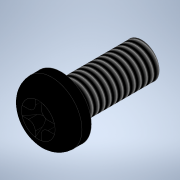
# Autodesk Inventor part: F-2606EB
Saved by Autodesk Inventor 2022.3 (Build 263350000, 350)
## iProperties
Part Number: F-2606EB
Material: チタン
Document SubType Name: Modeling
Designer: Masato Kubotera
Density: 6.22441 g/cm^3
Appearance: 陽極酸化 - 黒
Mass: 0.657 g
Surface Area: 1.94048 cm^2
Volume: 0.105552 cm^3
Description: ReadyMade
Catalog Web Link: https://wilco.jp/products/F/F-EB.html#page3
Author: Masato Kubotera
Autodesk Inventor part; units mm, degrees
ref_plane "YZ Plane" through (0, 0, 0) normal (1, 0, 0) x (0, 1, 0)
ref_plane "XZ Plane" through (0, 0, 0) normal (0, 1, 0) x (-1, 0, 0)
ref_plane "XY Plane" through (0, 0, 0) normal (0, 0, 1) x (1, 0, 0)
sketch "スケッチ1" plane through (0, 0, 0) normal (1, 0, 0) x (0, 1, 0)
  line L0 (0, 7.7) -> (0, 0)
  line L1 (0, 0) -> (1.25, 0)
  line L2 (2.25, 1) -> (2.25, 1.7)
  line L3 (2.25, 1.7) -> (1.3, 1.7)
  line L4 (1.3, 1.7) -> (1.3, 7.7)
  line L5 (1.3, 7.7) -> (0, 7.7)
  line L6 (1.25, 0) -> (0, 1.7)
  arc A0 (1.25, 0) -> (2.25, 1) centre (1.25, 1) ccw
  line L7 (1.25, 0) -> (2.25, 0)
  line L8 (2.25, 0) -> (2.25, 1)
  dimension "d2" = 1.7
  dimension "d10" = 6
  dimension "d11" = 2.6
  dimension "d12" = 4.5
  dimension "d14" = 1
  constraints: 18 end point, 6 perpendicular, 4 point on line, 2 point on circle, 2 tangent, 1 centre point, 1 horizontal, 1 vertical
  measures "d2" distance of L7.end L2.end
  measures "d10" distance of L3.end L4.end
  measures "d11" diameter of L4 L0
  measures "d12" diameter of L2 L0
  measures "d14" radius of A0
revolve "回転1" add sketch "スケッチ1" angle 360 about axis through (0, 0, 7.7) along (0, 0, -1) contours L5 L4 L3 L2 A0 L6 L0
thread "ねじ1" size "M2.6x0.45" class "6g" standard "ANSI Metric M Profile" full length
sketch "スケッチ2" plane through (0, 0, 1.7) normal (0, 0, 1) x (1, 0, 0)
  line L0 (0.3339, -1.6357) -> (-0.3339, -1.6357)
  line L1 (-0.3339, -1.6357) -> (-0.3339, -0.7226)
  line L2 (-0.3339, 1.6357) -> (0.3339, 1.6357)
  line L3 (0.3339, 1.6357) -> (0.3339, 0.7226)
  line L4 (0.3339, -1.6357) -> (-0.3339, 1.6357) construction
  line L5 (-0.3339, -1.6357) -> (0.3339, 1.6357) construction
  line L6 (-1.5922, 0.2226) -> (-0.8339, 0.2226)
  line L7 (1.5922, 0.2226) -> (1.5922, -0.2226)
  line L8 (1.5922, -0.2226) -> (0.8339, -0.2226)
  line L9 (-1.5922, -0.2226) -> (-1.5922, 0.2226)
  line L10 (-1.5922, 0.2226) -> (1.5922, -0.2226) construction
  line L11 (1.5922, 0.2226) -> (-1.5922, -0.2226) construction
  circle A0 centre (0, 0) radius 2.25
  line L12 (0.3339, -0.7226) -> (0.3339, -1.6357)
  line L13 (0.8339, 0.2226) -> (1.5922, 0.2226)
  line L14 (-0.8339, -0.2226) -> (-1.5922, -0.2226)
  line L15 (-0.3339, 0.7226) -> (-0.3339, 1.6357)
  arc A1 (0.8339, -0.2226) -> (0.3339, -0.7226) centre (0.8339, -0.7226) ccw
  arc A2 (0.3339, 0.7226) -> (0.8339, 0.2226) centre (0.8339, 0.7226) ccw
  arc A3 (-0.8339, 0.2226) -> (-0.3339, 0.7226) centre (-0.8339, 0.7226) ccw
  arc A4 (-0.3339, -0.7226) -> (-0.8339, -0.2226) centre (-0.8339, -0.7226) ccw
  point P0 (0, 0)
  point P1 (-0.3339, -0.2226)
  point P2 (-0.3339, 0.2226)
  point P3 (0.3339, 0.2226)
  point P4 (0.3339, -0.2226)
  dimension "d18" = 0.5
  constraints: 32 end point, 10 parallel, 8 point on circle, 8 tangent, 5 centre point, 4 midpoint, 4 perpendicular, 3 equal radius, 3 horizontal, 1 coincident
  measures "d18" radius of A1
extrude "押し出し2" add sketch "スケッチ2" against normal blind 1.7
revolve "回転2" cut sketch "スケッチ1" angle 360 about axis through (0, 0, 7.7) along (0, 0, -1) contours A0 L8 L7
